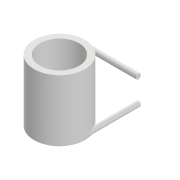
# Autodesk Inventor part: Torsion_spring
Saved by Autodesk Inventor 2022 (Build 260153000, 153)
## iProperties
Created: 2022-08-15
Part Number: Torsion_spring
Material: Generic
Document SubType Name: Modeling
Designer: dell
Density: 1 g/cm^3
Appearance: Stainless - Polished
Author: dell
Autodesk Inventor part; units mm, degrees
ref_plane "YZ Plane" through (0, 0, 0) normal (1, 0, 0) x (0, 1, 0)
ref_plane "XZ Plane" through (0, 0, 0) normal (0, 1, 0) x (-1, 0, 0)
ref_plane "XY Plane" through (0, 0, 0) normal (0, 0, 1) x (1, 0, 0)
sketch "Sketch1" plane through (0, 0, 0) normal (0, 1, 0) x (-1, 0, 0)
  circle A0 centre (0, 0) radius 4.55
  circle A1 centre (0, 0) radius 3.5
  dimension "d0" = 9.1
  dimension "d1" = 7
  constraints: 2 centre point, 2 coincident
  measures "d0" diameter of A0
  measures "d1" diameter of A1
extrude "Extrusion1" add sketch "Sketch1" along normal blind 11
sketch "Sketch2" plane through (0, 0, 0) normal (0, 0, 1) x (1, 0, 0)
  line L0 (4.55, 11) -> (-4.55, 11) projected
  line L1 (4.55, 0) -> (-4.55, 0) projected
  line L2 (4.55, 0) -> (-4.55, 0) projected
  line L3 (4.55, 0) -> (4.55, 11) projected
  line L4 (-4.55, 0) -> (-4.55, 11) projected
  circle A0 centre (4.1, 0.45) radius 0.45
  point P0 (0, 0)
  dimension "d11" = 0.9
  constraints: 2 tangent, 1 centre point
  measures "d11" diameter of A0
extrude "Extrusion2" add sketch "Sketch2" against normal blind 10 contours A0
sketch "Sketch3" plane through (0, 0, 0) normal (1, 0, 0) x (0, 1, 0)
  line L0 (0, -4.55) -> (0, 4.55) projected
  line L1 (11, -4.55) -> (11, 4.55) projected
  line L2 (11, -4.55) -> (11, 4.55) projected
  line L3 (0, 4.55) -> (11, 4.55) projected
  line L4 (0, -4.55) -> (11, -4.55) projected
  circle A0 centre (10.55, -4.1) radius 0.45
  point P0 (0, 0)
  point P1 (0, -1.9729)
  point P2 (0.45, 0)
  dimension "d12" = 0.9
  constraints: 2 tangent, 1 centre point, 2 other
  measures "d12" diameter of A0
extrude "Extrusion3" add sketch "Sketch3" along normal blind 10 contours A0
body "Solid1"
